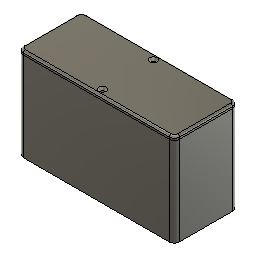
Fusion360_file (Autodesk Fusion 360 design; units mm, degrees)
Autodesk Fusion 360 part; units mm, degrees
sketch "Schizzo1" plane through (0, 0, 0) normal (0, 1, 0) x (1, 0, 0)
  line L0 (4, 0) -> (78, 0)
  line L1 (74, 64) -> (4, 64)
  line L2 (0, 60) -> (0, 4)
  circle A0 centre (74.05, 40.75) radius 1.3
  circle A1 centre (74.17, 12.95) radius 1.3
  circle A2 centre (22.07, 8) radius 1.3
  circle A3 centre (23.22, 55.9) radius 1.3
  line L3 (8, 58.78) -> (8, 5.44)
  arc A4 (4, 64) -> (0, 60) centre (4, 60) ccw
  arc A5 (0, 4) -> (4, 0) centre (4, 4) ccw
  line L4 (8, 47.1566) -> (8, 48.1566)
  line L5 (8, 48.1566) -> (0, 48.1566)
  line L6 (8, 35.1995) -> (8, 34.1995)
  line L7 (8, 34.1995) -> (0, 34.1995)
  line L8 (0, 48.1566) -> (-1.5, 48.1566)
  line L9 (0, 34.1995) -> (-1.5, 34.1995)
  line L10 (39, 32) -> (39, 64) construction
  line L11 (39, 32) -> (0, 32) construction
  circle A6 centre (19.5, 32) radius 3.85
  circle A7 centre (58.5, 32) radius 3.85
  line L12 (78, 0) -> (158, 0)
  line L13 (162, 4) -> (162, 60)
  line L14 (158, 64) -> (74, 64)
  arc A8 (162, 60) -> (158, 64) centre (158, 60) ccw
  arc A9 (158, 0) -> (162, 4) centre (158, 4) ccw
  line L15 (78, -1.5) -> (158, -1.5)
  arc A10 (158, -1.5) -> (163.5, 4) centre (158, 4) ccw
  line L16 (163.5, 4) -> (163.5, 60)
  arc A11 (163.5, 60) -> (158, 65.5) centre (158, 60) ccw
  line L17 (158, 65.5) -> (74, 65.5)
  line L18 (74, 65.5) -> (4, 65.5)
  arc A12 (4, 65.5) -> (-1.5, 60) centre (4, 60) ccw
  line L19 (-1.5, 60) -> (-1.5, 4)
  arc A13 (-1.5, 4) -> (4, -1.5) centre (4, 4) ccw
  line L20 (4, -1.5) -> (78, -1.5)
  line L21 (78, 0) -> (78, 64) construction
  circle A14 centre (97.5, 32) radius 3.85
  circle A15 centre (136.5, 32) radius 3.85
  point P0 (78, 0)
  point P1 (162, 0)
  dimension "d2" = 78
  dimension "d4" = 2.6
  dimension "d5" = 2.6
  dimension "d6" = 2.6
  dimension "d7" = 2.6
  dimension "d8" = 53.34
  dimension "d9" = 4
  dimension "d10" = 4
  dimension "d13" = 1
  dimension "d14" = 1
  dimension "d16" = 7.7
  dimension "d39" = 84
  dimension "d40" = 4
  dimension "d41" = 4
  dimension "d42" = 1.5
  constraint horizontal L0
  constraint perpendicular L0 L2
  constraint perpendicular L1 L3
  constraint tangent L2 A4
  constraint tangent L1 A4
  constraint coincident origin L0
  constraint tangent L2 A5
  constraint tangent L0 A5
  constraint coincident P0 L0
  constraint coincident L3 L4.start
  constraint coincident L3 L4.end
  constraint coincident L2 L5.end
  constraint perpendicular L2 L5
  constraint coincident L3 L6.start
  constraint coincident L3 L6.end
  constraint coincident L2 L7.end
  constraint perpendicular L2 L7
  constraint midpoint L2 L11.end
  constraint midpoint L1 L10.end
  constraint midpoint L11 A6.centre
  constraint symmetric L10 A6 A7
  constraint coincident P0 L0.end
  constraint perpendicular L2 L12
  constraint perpendicular L1 L13
  constraint perpendicular L2 L14
  constraint tangent L14 A8
  constraint tangent L13 A8
  constraint coincident P1 L13
  constraint coincident P1 L12
  constraint tangent L13 A9
  constraint tangent L12 A9
  constraint coincident L14 L21.end
  constraint perpendicular L14 L21
  constraint symmetric A6 L21 A15
  constraint symmetric A7 L21 A14
  measures "d2" distance of origin P0
  measures "d4" diameter of A0
  measures "d5" diameter of A1
  measures "d6" diameter of A2
  measures "d7" diameter of A3
  measures "d8" distance of L3.start L3.end
  measures "d9" radius of A4
  measures "d10" radius of A5
  measures "d13" distance of L4.start L4.end
  measures "d14" distance of L6.start L6.end
  measures "d16" diameter of A6
  measures "d39" distance of P0 P1
  measures "d40" radius of A8
  measures "d41" radius of A9
extrude "Estrusione1" add sketch "Schizzo1" against normal blind 4 contours L0 L1 L2 L3 A4 A5 L4 L5 L6 L7 L12 L13 L14 A8 A9 | L0 L1 L2 A4 A5 L8 L9 L12 L13 L14 A8 A9 L15 A10 L16 A11 L17 L18 A12 L19 A13 L20 | L2 L8 L9 L19 | L2 L3 L4 L5 L6 L7 | A0 | A1 | A2 | A3 | A6 | A7 | A14 | A15 makes body 1
extrude "Estrusione2" add sketch "Schizzo1" along normal blind 4 contours A0 | A1 | A2 | A3 bodies 1
fillet "Raccordo1" radius 1 4 edges at (72.838, 4, -40.2799) (72.958, 4, -12.4799) (20.858, 4, -7.5299) (22.008, 4, -55.4299) on bodies 1
fillet "Raccordo2" radius 0.5 4 edges at (72.838, 0, -41.2201) (72.958, 0, -13.4201) (20.858, 0, -8.4701) (22.008, 0, -56.3701) on bodies 1
hole "Foratura1" at (19.5, 0, -32) at (58.5, 0, -32) at (97.5, 0, -32) at (136.5, 0, -32) direction (0, -1, 0) diameter 4 depth 48 tip angle 118 countersink diameter 7.7 countersink angle 73 bodies 1
extrude "Estrusione3" add sketch "Schizzo1" along normal blind 90 contours L0 L1 L2 A4 A5 L8 L9 L12 L13 L14 A8 A9 L15 A10 L16 A11 L17 L18 A12 L19 A13 L20 bodies 1
extrude "Estrusione4" add sketch "Schizzo1" along normal blind 2 contours L2 L8 L9 L19 bodies 1
sketch "Schizzo4" plane through (0, 90, 0) normal (0, 1, 0) x (-1, 0, 0)
  line L0 (0, -34.1995) -> (1.5, -34.1995)
  line L1 (1.5, -34.1995) -> (1.5, -4)
  arc A0 (1.5, -4) -> (-4, 1.5) centre (-4, -4) ccw
  line L2 (-4, 1.5) -> (-158, 1.5)
  arc A1 (-158, 1.5) -> (-163.5, -4) centre (-158, -4) ccw
  line L3 (-163.5, -4) -> (-163.5, -60)
  arc A2 (-163.5, -60) -> (-158, -65.5) centre (-158, -60) ccw
  line L4 (-158, -65.5) -> (-4, -65.5)
  arc A3 (-4, -65.5) -> (1.5, -60) centre (-4, -60) ccw
  line L5 (1.5, -60) -> (1.5, -48.1566)
  line L6 (1.5, -48.1566) -> (0, -48.1566)
  line L7 (0, -48.1566) -> (0, -60)
  arc A4 (-4, -64) -> (0, -60) centre (-4, -60) ccw
  line L8 (-4, -64) -> (-158, -64)
  arc A5 (-162, -60) -> (-158, -64) centre (-158, -60) ccw
  line L9 (-162, -60) -> (-162, -4)
  arc A6 (-158, 0) -> (-162, -4) centre (-158, -4) ccw
  line L10 (-158, 0) -> (-4, 0)
  arc A7 (0, -4) -> (-4, 0) centre (-4, -4) ccw
  line L11 (0, -4) -> (0, -34.1995)
  line L12 (0, -60) -> (0, -4)
  line L13 (1.5, -60) -> (1.5, -4)
  line L14 (0, -48.1566) -> (1.5, -48.1566)
  line L15 (0, -34.1995) -> (1.5, -34.1995)
extrude "Estrusione7" add sketch "Schizzo4" against normal blind 77 contours L0 L6 L12 L13 L14 L15 bodies 1
sketch "Schizzo5" plane through (-1.5, 0, 0) normal (-1, 0, 0) x (0, 0, 1)
  line L0 (-34.1995, 13) -> (-34.1995, 2)
  line L1 (-34.1995, 2) -> (-48.1566, 2)
  line L2 (-48.1566, 2) -> (-48.1566, 13)
  line L3 (-48.1566, 13) -> (-34.1995, 13)
  line L4 (-4, 90) -> (-60, 90)
  line L5 (-60, 90) -> (-60, -4)
  line L6 (-60, -4) -> (-4, -4)
  line L7 (-4, -4) -> (-4, 90)
  line L8 (-49.1566, 1) -> (-49.1566, 14)
  line L9 (-49.1566, 14) -> (-33.1995, 14)
  line L10 (-33.1995, 14) -> (-33.1995, 1)
  line L11 (-33.1995, 1) -> (-49.1566, 1)
  line L12 (-60, 55) -> (-4, 55) construction
  line L13 (-32, 55) -> (-32, 65.25) construction
  line L14 (-32, 65.25) -> (-24.25, 65.25) construction
  line L15 (-24.25, 65.25) -> (-24.25, 44.75)
  line L16 (-24.25, 44.75) -> (-39.75, 44.75)
  line L17 (-39.75, 44.75) -> (-39.75, 65.25)
  line L18 (-39.75, 65.25) -> (-24.25, 65.25)
  line L19 (-4, 90) -> (-4, 82) construction
  line L20 (-4, 82) -> (-12, 82) construction
  circle A0 centre (-12, 82) radius 2.5
  dimension "d45" = -1
  dimension "d48" = 10.25
  dimension "d49" = 7.75
  dimension "d50" = 20.5
  dimension "d51" = 15.5
  dimension "d95" = 5
  constraint coincident L5 L12.start
  constraint coincident L7 L12.end
  constraint perpendicular L7 L12
  constraint midpoint L12 L13.start
  constraint perpendicular L12 L13
  constraint perpendicular L13 L14
  constraint perpendicular L12 L15
  constraint perpendicular L5 L16
  constraint perpendicular L14 L17
  constraint perpendicular L15 L18
  constraint coincident L4.start L7.end
  constraint coincident L7 L19.end
  constraint perpendicular L4 L19
  constraint perpendicular L7 L20
  constraint coincident L20.end A0.centre
  measures "d48" distance of L13.start L13.end
  measures "d49" distance of L13.end L14.end
  measures "d50" distance of L14.end L15.end
  measures "d51" distance of L15.end L16.end
  measures "d95" diameter of A0
extrude "Estrusione8" cut sketch "Schizzo5" against normal blind 5 contours L8 L9 L10 L11 bodies 1
extrude "Estrusione10" cut sketch "Schizzo5" against normal blind 15 contours L15 L16 L17 L18 bodies 1
ref_plane "Piano di lavoro1" through (81, 90, -32) normal (0, 1, 0) x (1, 0, 0)
sketch "Schizzo7" plane through (0, 0, -64) normal (0, 0, 1) x (1, 0, 0)
  line L0 (4, 0) -> (158, 0)
  line L1 (158, 0) -> (158, 90)
  line L2 (158, 90) -> (4, 90)
  line L3 (4, 90) -> (4, 0)
  line L4 (81, 90) -> (81, 80) construction
  line L5 (81, 80) -> (71, 80)
  line L6 (71, 80) -> (71, 90)
  line L7 (81, 80) -> (91, 80)
  line L8 (91, 80) -> (91, 90)
  line L9 (71, 80) -> (81, 70)
  line L10 (71, 80) -> (85.1421, 80) construction
  line L11 (81, 70) -> (91, 80)
  dimension "d57" = 45
  constraint midpoint L2 L4.start
  constraint perpendicular L2 L4
  constraint perpendicular L4 L5
  constraint coincident L2 L6.end
  constraint perpendicular L2 L6
  constraint symmetric L5.start L4 L7.start
  constraint symmetric L4 L5.end L7.end
  constraint symmetric L4 L6.end L8.end
  constraint horizontal L10
  constraint perpendicular L9 L11
  measures "d57" angle of L9 L10
extrude "Estrusione11" add sketch "Schizzo7" along normal blind 10 contours L2 L5 L6 L7 L8 | L5 L7 L9 L11 bodies 1
sketch "Schizzo8" plane through (71, 0, 0) normal (-1, 0, 0) x (0, 0, 1)
  line L0 (-64, 90) -> (-64, 80)
  line L1 (-64, 80) -> (-54, 80)
  line L2 (-54, 80) -> (-54, 90)
  line L3 (-54, 90) -> (-64, 90)
  line L4 (-64, 80) -> (-64, 70)
  line L5 (-64, 70) -> (-54, 70)
  line L6 (-54, 70) -> (-54, 80)
  line L7 (-54, 80) -> (-64, 80)
  line L8 (-64, 70) -> (-54, 80)
  constraint coincident L4.end L5.start
  constraint coincident L1.end L2.start
extrude "Estrusione12" cut sketch "Schizzo8" against normal blind 25 contours L5 L6 L8 bodies 1
sketch "Schizzo9" plane through (0, 90, 0) normal (0, 1, 0) x (-1, 0, 0)
  line L0 (1.5, -60) -> (1.5, -4)
  arc A0 (1.5, -4) -> (-4, 1.5) centre (-4, -4) ccw
  line L1 (-4, 1.5) -> (-158, 1.5)
  arc A1 (-158, 1.5) -> (-163.5, -4) centre (-158, -4) ccw
  line L2 (-163.5, -4) -> (-163.5, -60)
  arc A2 (-163.5, -60) -> (-158, -65.5) centre (-158, -60) ccw
  line L3 (-158, -65.5) -> (-4, -65.5)
  arc A3 (-4, -65.5) -> (1.5, -60) centre (-4, -60) ccw
  line L4 (0, -4) -> (0, -60)
  arc A4 (-4, -64) -> (0, -60) centre (-4, -60) ccw
  line L5 (-4, -64) -> (-71, -64)
  line L6 (-71, -64) -> (-71, -54)
  line L7 (-71, -54) -> (-91, -54)
  line L8 (-91, -54) -> (-91, -64)
  line L9 (-91, -64) -> (-158, -64)
  arc A5 (-162, -60) -> (-158, -64) centre (-158, -60) ccw
  line L10 (-162, -60) -> (-162, -4)
  arc A6 (-158, 0) -> (-162, -4) centre (-158, -4) ccw
  line L11 (-158, 0) -> (-4, 0)
  arc A7 (0, -4) -> (-4, 0) centre (-4, -4) ccw
  line L12 (-71, -59) -> (-91, -59) construction
  line L13 (-81, -54) -> (-81, -64) construction
  circle A8 centre (-81, -59) radius 1.85
  line L14 (-71, -64) -> (-91, -64)
  line L15 (-71, -64) -> (-71, -54)
  line L16 (-91, -54) -> (-91, -64)
  line L17 (-91, -54) -> (-71, -54)
  dimension "d62" = 3.7
  constraint midpoint L6 L12.start
  constraint midpoint L8 L12.end
  constraint midpoint L7 L13.start
  constraint perpendicular L9 L13
  constraint midpoint L12 A8.centre
  constraint coincident L5.end L6.start
  constraint coincident L8.end L9.start
  constraint coincident L6.end L7.start
  constraint coincident L7.end L8.start
  measures "d62" diameter of A8
ref_plane "Piano di lavoro2" through (81, 45, -32) normal (0, 0, 1) x (1, 0, 0)
extrude "Estrusione13" add 1 faces at (84.3333, 90, -57.3333) along direction (0, 1, 0) blind 2 on bodies 1 bodies 1
split "Dividi1" by plane through (81, 90, -32) normal (0, 1, 0) bodies 1 makes body 2 at (84.3333, 92, -57.3333)
extrude "Estrusione16" cut sketch "Schizzo9" against normal blind 22 contours A8 bodies 1
mirror "Specchio3" about plane through (81, 45, -32) normal (0, 0, 1) of 7 faces at (84.3333, 83.3333, -54) (71, 83.3333, -60.6667) (91, 83.3333, -60.6667) (87.6667, 76.6667, -60.6667) (79.1623, 79.8796, -59.213) (81.0262, 78.9494, -55.0506) (74.3333, 76.6667, -60.6667) on bodies 1
delete_body "RimuoviCorpo2" bodies 2
extrude "Estrusione17" add 1 faces at (88.2805, 90, -59.0586) along direction (0, 1, 0) blind 4 on bodies 1 bodies 1
split "Dividi2" by plane through (81, 90, -32) normal (0, 1, 0) bodies 1 makes body 3 at (88.2805, 94, -59.0586)
sketch "Schizzo11" plane through (0, 94, 0) normal (0, 1, 0) x (-1, 0, 0)
  circle A0 centre (-81, -59) radius 1.85
  line L0 (-91, 0) -> (-91, -10)
  line L1 (-91, -10) -> (-71, -10)
  line L2 (-71, -10) -> (-71, 0)
  line L3 (-71, 0) -> (-4, 0)
  arc A1 (0, -4) -> (-4, 0) centre (-4, -4) ccw
  line L4 (0, -4) -> (0, -60)
  arc A2 (-4, -64) -> (0, -60) centre (-4, -60) ccw
  line L5 (-4, -64) -> (-71, -64)
  line L6 (-71, -64) -> (-71, -54)
  line L7 (-71, -54) -> (-91, -54)
  line L8 (-91, -54) -> (-91, -64)
  line L9 (-91, -64) -> (-158, -64)
  arc A3 (-162, -60) -> (-158, -64) centre (-158, -60) ccw
  line L10 (-162, -60) -> (-162, -4)
  arc A4 (-158, 0) -> (-162, -4) centre (-158, -4) ccw
  line L11 (-158, 0) -> (-91, 0)
  line L12 (-4, 1.5) -> (-158, 1.5)
  arc A5 (-158, 1.5) -> (-163.5, -4) centre (-158, -4) ccw
  line L13 (-163.5, -4) -> (-163.5, -60)
  arc A6 (-163.5, -60) -> (-158, -65.5) centre (-158, -60) ccw
  line L14 (-158, -65.5) -> (-4, -65.5)
  arc A7 (-4, -65.5) -> (1.5, -60) centre (-4, -60) ccw
  line L15 (1.5, -60) -> (1.5, -4)
  arc A8 (1.5, -4) -> (-4, 1.5) centre (-4, -4) ccw
  circle A9 centre (-81, -5) radius 1.85
  line L16 (-70.6, -53.6) -> (-91.4, -53.6)
  line L17 (-91.4, -53.6) -> (-91.4, -63.6)
  line L18 (-91.4, -63.6) -> (-158, -63.6)
  arc A10 (-161.6, -60) -> (-158, -63.6) centre (-158, -60) ccw
  line L19 (-161.6, -60) -> (-161.6, -4)
  arc A11 (-158, -0.4) -> (-161.6, -4) centre (-158, -4) ccw
  line L20 (-158, -0.4) -> (-91.4, -0.4)
  line L21 (-91.4, -0.4) -> (-91.4, -10.4)
  line L22 (-91.4, -10.4) -> (-70.6, -10.4)
  line L23 (-70.6, -10.4) -> (-70.6, -0.4)
  line L24 (-70.6, -0.4) -> (-4, -0.4)
  arc A12 (-0.4, -4) -> (-4, -0.4) centre (-4, -4) ccw
  line L25 (-0.4, -4) -> (-0.4, -60)
  arc A13 (-4, -63.6) -> (-0.4, -60) centre (-4, -60) ccw
  line L26 (-4, -63.6) -> (-70.6, -63.6)
  line L27 (-70.6, -63.6) -> (-70.6, -53.6)
  dimension "d85" = 0.4
extrude "Estrusione18" add sketch "Schizzo11" against normal blind 4 contours L0 L1 L2 L3 A1 L4 A2 L5 L6 L7 L8 L9 A3 L10 A4 L11 | L12 A5 L13 A6 L14 A7 L15 A8 | L16 L17 L18 A10 L19 A11 L20 L21 L22 L23 L24 A12 L25 A13 L26 L27 bodies 3
extrude "Estrusione19" add sketch "Schizzo11" against normal blind 5 contours L16 L17 L18 A10 L19 A11 L20 L21 L22 L23 L24 A12 L25 A13 L26 L27 bodies 3
hole "Foratura3" at (81, 94, -59) at (81, 94, -5) direction (0, -1, 0) diameter 3.8 depth 18 tip angle 118 countersink diameter 7.7 countersink angle 73 bodies 3
extrude "Estrusione20" cut sketch "Schizzo5" against normal blind 2 contours A0 bodies 1
fillet "Raccordo3" radius 2 8 edges at (81, 94, 1.5) (161.8891, 94, -0.1109) (163.5, 94, -32) (161.8891, 94, -63.8891) (81, 94, -65.5) (0.1109, 94, -63.8891) (-1.5, 94, -32) (0.1109, 94, -0.1109) on bodies 3
named bodies: "Base", "Coperchio"
